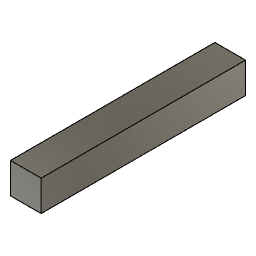
vesa_mount v7 (Autodesk Fusion 360 archive; units mm, degrees)
design "3030_profile"
Autodesk Fusion 360 part; units mm, degrees
sketch "Sketch1" plane through (0, 0, 0) normal (0, 1, 0) x (1, 0, 0)
  line L0 (-15, -15) -> (15, -15)
  line L1 (15, -15) -> (15, 15)
  line L2 (15, 15) -> (-15, 15)
  line L3 (-15, 15) -> (-15, -15)
  dimension "d1" = 30
  dimension "d2" = 30
  dimension "d3" = 15
  dimension "d4" = 15
  constraint horizontal L0
  constraint vertical L1
  constraint horizontal L2
  constraint vertical L3
  measures "d1" distance of L0.start L0.end
  measures "d2" distance of L0.start L2.end
  measures "d3" distance of origin L3
  measures "d4" distance of origin L0
extrude "Extrude1" add sketch "Sketch1" along normal blind 100 and the other way blind 100
